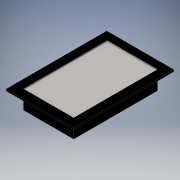
# Autodesk Inventor part: Computer
Saved by Autodesk Inventor 2016 (Build 200138000, 138)
## iProperties
Created: 2015-11-30
Part Number: Computer
Material: Generic
Document SubType Name: Modeling
Designer: Javier
Density: 1 g/cm^3
Appearance: Default
Author: Javier
Autodesk Inventor part; units mm, degrees
ref_plane "YZ Plane" through (0, 0, 0) normal (1, 0, 0) x (0, 1, 0)
ref_plane "XY Plane" through (0, 0, 0) normal (0, 0, 1) x (1, 0, 0)
sketch "Sketch1" plane through (0, 0, 0) normal (0, 1, 0) x (-1, 0, 0)
  line L0 (60.96, -81.28) -> (-40.64, -81.28)
  line L1 (-40.64, -81.28) -> (-40.64, 71.12)
  line L2 (-40.64, 71.12) -> (60.96, 71.12)
  line L3 (60.96, 71.12) -> (60.96, -81.28)
  point P0 (0, 0)
  dimension "d0" = 152.4
  dimension "d1" = 101.6
  constraints: 8 end point, 2 parallel, 1 horizontal, 1 perpendicular
  measures "d0" distance of L2.end L0.start
  measures "d1" distance between parallel lines of L1 L3
extrude "Extrusion1" add sketch "Sketch1" along normal blind 2.54
sketch "Sketch2" plane through (0, 0, 0) normal (0, 1, 0) x (-1, 0, 0)
  line L0 (48.26, 57.7273) -> (-27.94, 57.7273)
  line L1 (-27.94, 57.7273) -> (-27.94, -69.2727)
  line L2 (-27.94, -69.2727) -> (48.26, -69.2727)
  line L3 (48.26, -69.2727) -> (48.26, 57.7273)
  line L4 (60.96, -81.28) -> (60.96, 71.12) projected
  line L5 (-40.64, 71.12) -> (-40.64, -81.28) projected
  point P0 (0, 0)
  dimension "d4" = 127
  dimension "d5" = 76.2
  dimension "d11" = 12.7
  constraints: 8 end point, 2 parallel, 1 horizontal, 1 perpendicular
  measures "d4" distance between parallel lines of L2 L0
  measures "d5" distance between parallel lines of L1 L3
  measures "d11" distance between parallel lines of L3 L4
extrude "Extrusion2" add sketch "Sketch2" against normal blind 25.4
ref_plane "Work Plane1" through (0, 2.54, 0) normal (0, 1, 0) x (-1, 0, 0)
sketch "Sketch3" plane through (0, 2.54, 0) normal (0, 1, 0) x (-1, 0, 0)
  line L0 (48.26, 57.7273) -> (48.26, -69.2727) projected
  line L1 (-27.94, -69.2727) -> (-27.94, 57.7273) projected
  line L2 (48.26, 57.7273) -> (-27.94, 57.7273)
  line L3 (-27.94, 57.7273) -> (-27.94, -69.2727)
  line L4 (-27.94, -69.2727) -> (48.26, -69.2727)
  line L5 (48.26, -69.2727) -> (48.26, 57.7273)
  point P0 (0, 0)
  constraints: 8 end point, 2 parallel, 1 horizontal, 1 perpendicular
extrude "Extrusion3" cut sketch "Sketch3" against normal blind 1.27
body "Solid1"
